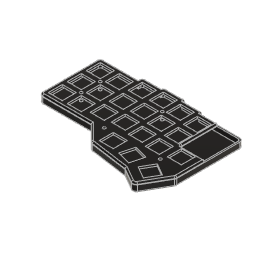
case-compact (Autodesk Fusion 360 design; units mm, degrees)
Autodesk Fusion 360 part; units mm, degrees
sketch "top_plate" plane through (0, 0, 0) normal (0, 0, 1) x (1, 0, 0)
  arc A0 (37, 57) -> (38, 58) centre (37, 58) ccw
  circle A1 centre (19, 38) radius 1.4
  circle A2 centre (76, 43) radius 1.4
  line L0 (117.5, 20.5) -> (131.5, 20.5)
  arc A3 (114, 24.5) -> (115.5, 23) centre (115.5, 24.5) ccw
  line L1 (95, 60) -> (95, 60)
  line L2 (95, 60) -> (95, 60)
  line L3 (96, 59) -> (112.5, 59)
  arc A4 (66.595, -15.7544) -> (67.4469, -16.1791) centre (67.6556, -14.6937) ccw
  line L4 (123.2697, -29.8066) -> (136.7998, -6.3468)
  arc A5 (106.318, -21.7524) -> (105.7767, -21.566) centre (105.568, -23.0514) ccw
  circle A6 centre (19, 19) radius 1.4
  line L5 (131.5, 20.5) -> (131.5, 6.5)
  line L6 (111.6878, -16.8122) -> (118.6878, -4.6878)
  line L7 (57, 62) -> (57, 62)
  arc A7 (0, 1.5) -> (1.5, 0) centre (1.5, 1.5) ccw
  line L8 (69.5, -13.5) -> (69.5, 0.5)
  line L9 (121.2203, -30.3563) -> (106.318, -21.7524)
  line L10 (118.6878, -4.6878) -> (130.8122, -11.6878)
  line L11 (58, 63) -> (75, 63)
  line L12 (38, 58) -> (38, 60)
  circle A8 centre (61, 0) radius 1.4
  line L13 (1.5, 57) -> (37, 57)
  line L14 (66.595, -15.7544) -> (51.2799, -0.4393)
  line L15 (93.5503, -0.9268) -> (107.0732, -4.5503)
  arc A9 (1.5, 57) -> (0, 55.5) centre (1.5, 55.5) ccw
  arc A10 (95, 60) -> (96, 59) centre (96, 60) ccw
  line L16 (117.5, 6.5) -> (117.5, 20.5)
  line L17 (135.5004, 23) -> (115.5, 23)
  line L18 (114, 24.5) -> (114, 57.5)
  arc A11 (121.2203, -30.3563) -> (123.2697, -29.8066) centre (121.9703, -29.0572) ccw
  arc A12 (136.7998, -6.3468) -> (137.0004, -5.5974) centre (135.5004, -5.5974) ccw
  arc A13 (76, 62) -> (75, 63) centre (75, 62) ccw
  line L19 (105.7767, -21.566) -> (67.4469, -16.1791)
  line L20 (123.8122, -23.8122) -> (111.6878, -16.8122)
  arc A14 (56, 61) -> (57, 62) centre (56, 62) ccw
  line L21 (0, 55.5) -> (0, 1.5)
  arc A15 (58, 63) -> (57, 62) centre (58, 62) ccw
  circle A16 centre (116, 1) radius 1.4
  arc A17 (39, 61) -> (38, 60) centre (39, 60) ccw
  line L22 (76, 62) -> (76, 62)
  line L23 (57, 62) -> (57, 62)
  line L24 (107.0732, -4.5503) -> (103.4497, -18.0732)
  line L25 (103.4497, -18.0732) -> (89.9268, -14.4497)
  line L26 (137.0004, 21.5) -> (137.0004, -5.5974)
  arc A18 (76, 62) -> (77, 61) centre (77, 62) ccw
  line L27 (89.9268, -14.4497) -> (93.5503, -0.9268)
  line L28 (76, 62) -> (76, 62)
  line L29 (1.5, 0) -> (50.2193, 0)
  line L30 (2.5, 40.5) -> (16.5, 40.5)
  line L31 (16.5, 40.5) -> (16.5, 54.5)
  line L32 (2.5, 54.5) -> (2.5, 40.5)
  line L33 (21.5, 2.5) -> (35.5, 2.5)
  line L34 (16.5, 35.5) -> (2.5, 35.5)
  line L35 (35.5, 2.5) -> (35.5, 16.5)
  line L36 (35.5, 21.5) -> (35.5, 35.5)
  line L37 (21.5, 16.5) -> (21.5, 2.5)
  line L38 (16.5, 54.5) -> (2.5, 54.5)
  line L39 (16.5, 21.5) -> (16.5, 35.5)
  line L40 (35.5, 16.5) -> (21.5, 16.5)
  line L41 (2.5, 35.5) -> (2.5, 21.5)
  line L42 (21.5, 21.5) -> (35.5, 21.5)
  line L43 (35.5, 35.5) -> (21.5, 35.5)
  line L44 (69.5, 0.5) -> (83.5, 0.5)
  line L45 (2.5, 21.5) -> (16.5, 21.5)
  line L46 (111.5, 42.5) -> (97.5, 42.5)
  line L47 (59.5, 8.5) -> (59.5, 22.5)
  line L48 (111.5, 37.5) -> (111.5, 23.5)
  line L49 (73.5, 46.5) -> (59.5, 46.5)
  line L50 (73.5, 41.5) -> (73.5, 27.5)
  line L51 (73.5, 22.5) -> (73.5, 8.5)
  line L52 (97.5, 18.5) -> (111.5, 18.5)
  line L53 (92.5, 39.5) -> (78.5, 39.5)
  line L54 (40.5, 20.5) -> (40.5, 6.5)
  line L55 (59.5, 27.5) -> (59.5, 41.5)
  line L56 (111.5, 4.5) -> (97.5, 4.5)
  line L57 (54.5, 44.5) -> (54.5, 58.5)
  line L58 (54.5, 20.5) -> (40.5, 20.5)
  line L59 (16.5, 2.5) -> (16.5, 16.5)
  line L60 (40.5, 39.5) -> (40.5, 25.5)
  line L61 (21.5, 40.5) -> (35.5, 40.5)
  line L62 (97.5, 56.5) -> (111.5, 56.5)
  line L63 (59.5, 60.5) -> (73.5, 60.5)
  line L64 (40.5, 44.5) -> (54.5, 44.5)
  line L65 (111.5, 56.5) -> (111.5, 42.5)
  line L66 (40.5, 25.5) -> (54.5, 25.5)
  line L67 (35.5, 40.5) -> (35.5, 54.5)
  arc A19 (95, 60) -> (94, 61) centre (94, 60) ccw
  line L68 (97.5, 23.5) -> (97.5, 37.5)
  line L69 (35.5, 54.5) -> (21.5, 54.5)
  line L70 (78.5, 39.5) -> (78.5, 25.5)
  line L71 (59.5, 22.5) -> (73.5, 22.5)
  line L72 (92.5, 44.5) -> (92.5, 58.5)
  line L73 (111.5, 23.5) -> (97.5, 23.5)
  line L74 (92.5, 25.5) -> (92.5, 39.5)
  line L75 (131.5, 6.5) -> (117.5, 6.5)
  line L76 (97.5, 4.5) -> (97.5, 18.5)
  line L77 (54.5, 58.5) -> (40.5, 58.5)
  line L78 (83.5, 0.5) -> (83.5, -13.5)
  line L79 (73.5, 8.5) -> (59.5, 8.5)
  line L80 (111.5, 18.5) -> (111.5, 4.5)
  line L81 (21.5, 35.5) -> (21.5, 21.5)
  line L82 (92.5, 6.5) -> (92.5, 20.5)
  line L83 (16.5, 16.5) -> (2.5, 16.5)
  line L84 (59.5, 41.5) -> (73.5, 41.5)
  line L85 (78.5, 6.5) -> (92.5, 6.5)
  line L86 (40.5, 58.5) -> (40.5, 44.5)
  line L87 (92.5, 20.5) -> (78.5, 20.5)
  line L88 (54.5, 25.5) -> (54.5, 39.5)
  line L89 (2.5, 16.5) -> (2.5, 2.5)
  line L90 (73.5, 27.5) -> (59.5, 27.5)
  line L91 (78.5, 25.5) -> (92.5, 25.5)
  line L92 (54.5, 6.5) -> (54.5, 20.5)
  line L93 (92.5, 58.5) -> (78.5, 58.5)
  arc A20 (137.0004, 21.5) -> (135.5004, 23) centre (135.5004, 21.5) ccw
  line L94 (130.8122, -11.6878) -> (123.8122, -23.8122)
  line L95 (39, 61) -> (56, 61)
  line L96 (77, 61) -> (94, 61)
  line L97 (40.5, 6.5) -> (54.5, 6.5)
  arc A21 (114, 57.5) -> (112.5, 59) centre (112.5, 57.5) ccw
  line L98 (97.5, 42.5) -> (97.5, 56.5)
  line L99 (78.5, 44.5) -> (92.5, 44.5)
  line L100 (21.5, 54.5) -> (21.5, 40.5)
  line L101 (73.5, 60.5) -> (73.5, 46.5)
  line L102 (59.5, 46.5) -> (59.5, 60.5)
  line L103 (54.5, 39.5) -> (40.5, 39.5)
  line L104 (78.5, 58.5) -> (78.5, 44.5)
  arc A22 (51.2799, -0.4393) -> (50.2193, 0) centre (50.2193, -1.5) ccw
  line L105 (97.5, 37.5) -> (111.5, 37.5)
  line L106 (83.5, -13.5) -> (69.5, -13.5)
  line L107 (2.5, 2.5) -> (16.5, 2.5)
  line L108 (78.5, 20.5) -> (78.5, 6.5)
  line L109 (77.8284, 63) -> (94, 63)
  arc A23 (96.8284, 61) -> (94, 63) centre (94, 60) ccw
  line L110 (96.8284, 61) -> (112.5, 61)
  line L111 (139.0004, 21.5) -> (139.0004, -5.5974)
  arc A24 (138.5323, -7.346) -> (139.0004, -5.5974) centre (135.5004, -5.5974) ccw
  line L112 (125.0022, -30.8058) -> (138.5323, -7.346)
  arc A25 (120.2203, -32.0883) -> (125.0022, -30.8058) centre (121.9703, -29.0572) ccw
  line L113 (120.2203, -32.0883) -> (105.4021, -23.5331)
  line L114 (105.4021, -23.5331) -> (67.1685, -18.1597)
  arc A26 (65.1808, -17.1686) -> (67.1685, -18.1597) centre (67.6556, -14.6937) ccw
  line L115 (65.1808, -17.1686) -> (50.0122, -2)
  line L116 (1.5, -2) -> (50.0122, -2)
  arc A27 (-2, 1.5) -> (1.5, -2) centre (1.5, 1.5) ccw
  line L117 (-2, 55.5) -> (-2, 1.5)
  arc A28 (1.5, 59) -> (-2, 55.5) centre (1.5, 55.5) ccw
  line L118 (1.5, 59) -> (36, 59)
  line L119 (36, 59) -> (36, 60)
  arc A29 (39, 63) -> (36, 60) centre (39, 60) ccw
  line L120 (39, 63) -> (55.1716, 63)
  arc A30 (58, 65) -> (55.1716, 63) centre (58, 62) ccw
  line L121 (58, 65) -> (75, 65)
  arc A31 (77.8284, 63) -> (75, 65) centre (75, 62) ccw
  line L122 (114, 57.5) -> (114, 59.5)
  line L123 (135.5004, 23) -> (137.5004, 23)
  arc A32 (114, 59.5) -> (112.5, 61) centre (112.5, 59.5) ccw
  arc A33 (139.0004, 21.5) -> (137.5004, 23) centre (137.5004, 21.5) ccw
  dimension "d10" = 1.5
  dimension "d11" = 1.5
  constraint tangent A21 L122
  constraint perpendicular L110 L122
  constraint parallel L96 L109
  constraint concentric A19 A23
  constraint parallel L3 L110
  constraint parallel L26 L111
  constraint concentric A12 A24
  constraint parallel L4 L112
  constraint concentric A11 A25
  constraint parallel L9 L113
  constraint parallel L19 L114
  constraint concentric A4 A26
  constraint parallel L14 L115
  constraint parallel L29 L116
  constraint concentric A7 A27
  constraint parallel L21 L117
  constraint concentric A9 A28
  constraint parallel L13 L118
  constraint parallel L12 L119
  constraint concentric A17 A29
  constraint parallel L95 L120
  constraint concentric A15 A30
  constraint parallel L11 L121
  constraint concentric A13 A31
  constraint tangent L109 A23
  constraint tangent A29 L120
  constraint tangent L111 A24
  constraint tangent A24 L112
  constraint tangent L112 A25
  constraint tangent A25 L113
  constraint tangent L114 A26
  constraint tangent A26 L115
  constraint tangent L116 A27
  constraint tangent A27 L117
  constraint tangent L117 A28
  constraint tangent A28 L118
  constraint tangent L119 A29
  constraint tangent A30 L121
  constraint tangent L121 A31
  constraint tangent A20 L123
  constraint perpendicular L111 L123
  constraint tangent L110 A32
  constraint tangent L122 A32
  constraint tangent L123 A33
  constraint tangent L111 A33
  measures "d10" radius of A32
  measures "d11" radius of A33
extrude "Extrude4" add sketch "top_plate" along normal blind 2 makes body 1
fillet "Fillet1" radius 1.5 27 edges at (18.75, 59, 2) (-0.9749, 57.9749, 2) (-2, 28.5, 2) (-0.9749, -0.9749, 2) (25.7561, -2, 2) (57.5965, -9.5843, 2) (66.0939, -17.826, 2) (86.2853, -20.8464, 2) (112.8112, -27.8107, 2) (122.8769, -32.4378, 2) (131.7673, -19.0759, 2) (138.8814, -6.5025, 2) (139.0004, 7.9513, 2) (138.5611, 22.5607, 2) (126.5002, 23, 2) (114.4393, 23.4393, 2) (114, 42, 2) (113.5607, 60.5607, 2) (104.6642, 61, 2) (95.7321, 62.4495, 2) (85.9142, 63, 2) (76.7321, 64.4495, 2) (66.5, 65, 2) (56.2679, 64.4495, 2) (47.0858, 63, 2) (36.8787, 62.1213, 2) (36, 59.5, 2) on bodies 1
sketch "bottom_plate" plane through (0, 0, 0) normal (0, 0, 1) x (1, 0, 0) in component "case-bottom"
  circle A0 centre (19, 38) radius 1.4
  circle A1 centre (61, 0) radius 1.4
  circle A2 centre (116, 1) radius 1.4
  arc A3 (56, 61) -> (57, 62) centre (56, 62) ccw
  circle A4 centre (76, 43) radius 1.4
  line L0 (121.2203, -30.3563) -> (106.318, -21.7524)
  line L1 (76, 62) -> (76, 62)
  line L2 (57, 62) -> (57, 62)
  line L3 (105.7767, -21.566) -> (67.4469, -16.1791)
  arc A5 (121.2203, -30.3563) -> (123.2697, -29.8066) centre (121.9703, -29.0572) ccw
  arc A6 (136.7994, -6.3479) -> (137, -5.5984) centre (135.5, -5.5984) ccw
  arc A7 (106.318, -21.7524) -> (105.7767, -21.566) centre (105.568, -23.0514) ccw
  arc A8 (76, 62) -> (75, 63) centre (75, 62) ccw
  line L4 (58, 63) -> (75, 63)
  arc A9 (95, 60) -> (96, 59) centre (96, 60) ccw
  arc A10 (0, 1.5) -> (1.5, 0) centre (1.5, 1.5) ccw
  arc A11 (51.2799, -0.4393) -> (50.2193, 0) centre (50.2193, -1.5) ccw
  line L5 (123.2697, -29.8066) -> (136.7994, -6.3479)
  arc A12 (37, 57) -> (38, 58) centre (37, 58) ccw
  arc A13 (66.595, -15.7544) -> (67.4469, -16.1791) centre (67.6556, -14.6937) ccw
  line L6 (1.5, 0) -> (50.2193, 0)
  line L7 (38, 58) -> (38, 60)
  line L8 (76, 62) -> (76, 62)
  line L9 (39, 61) -> (56, 61)
  arc A14 (39, 61) -> (38, 60) centre (39, 60) ccw
  line L10 (95, 60) -> (95, 60)
  line L11 (95, 60) -> (95, 60)
  line L12 (66.595, -15.7544) -> (51.2799, -0.4393)
  line L13 (0, 55.5) -> (0, 1.5)
  line L14 (1.5, 57) -> (37, 57)
  arc A15 (1.5, 57) -> (0, 55.5) centre (1.5, 55.5) ccw
  line L15 (77, 61) -> (94, 61)
  line L16 (57, 62) -> (57, 62)
  arc A16 (58, 63) -> (57, 62) centre (58, 62) ccw
  circle A17 centre (19, 19) radius 1.4
  line L17 (137, 57.5) -> (137, -5.5984)
  arc A18 (137, 57.5) -> (135.5, 59) centre (135.5, 57.5) ccw
  arc A19 (76, 62) -> (77, 61) centre (77, 62) ccw
  line L18 (95, 60) -> (95, 60)
  arc A20 (95, 60) -> (94, 61) centre (94, 60) ccw
  line L19 (96, 59) -> (135.5, 59)
  line L20 (96.8284, 61) -> (135.5, 61)
  arc A21 (139, 57.5) -> (135.5, 61) centre (135.5, 57.5) ccw
  line L21 (139, 57.5) -> (139, -5.5984)
  arc A22 (138.5319, -7.3471) -> (139, -5.5984) centre (135.5, -5.5984) ccw
  line L22 (125.0022, -30.8059) -> (138.5319, -7.3471)
  arc A23 (120.2203, -32.0883) -> (125.0022, -30.8059) centre (121.9703, -29.0572) ccw
  line L23 (120.2203, -32.0883) -> (105.4021, -23.5331)
  line L24 (105.4021, -23.5331) -> (67.1685, -18.1597)
  arc A24 (65.1808, -17.1686) -> (67.1685, -18.1597) centre (67.6556, -14.6937) ccw
  line L25 (65.1808, -17.1686) -> (50.0122, -2)
  line L26 (1.5, -2) -> (50.0122, -2)
  arc A25 (-2, 1.5) -> (1.5, -2) centre (1.5, 1.5) ccw
  line L27 (-2, 55.5) -> (-2, 1.5)
  arc A26 (1.5, 59) -> (-2, 55.5) centre (1.5, 55.5) ccw
  line L28 (1.5, 59) -> (36, 59)
  line L29 (36, 59) -> (36, 60)
  arc A27 (39, 63) -> (36, 60) centre (39, 60) ccw
  line L30 (39, 63) -> (55.1716, 63)
  arc A28 (58, 65) -> (55.1716, 63) centre (58, 62) ccw
  line L31 (58, 65) -> (75, 65)
  arc A29 (77.8284, 63) -> (75, 65) centre (75, 62) ccw
  line L32 (77.8284, 63) -> (94, 63)
  arc A30 (96.8284, 61) -> (94, 63) centre (94, 60) ccw
  arc A31 (95.5, 60) -> (96, 59.5) centre (96, 60) ccw
  line L33 (96, 59.5) -> (135.5, 59.5)
  arc A32 (137.5, 57.5) -> (135.5, 59.5) centre (135.5, 57.5) ccw
  line L34 (137.5, 57.5) -> (137.5, -5.5984)
  arc A33 (137.2325, -6.5977) -> (137.5, -5.5984) centre (135.5, -5.5984) ccw
  line L35 (123.7028, -30.0564) -> (137.2325, -6.5977)
  arc A34 (120.9703, -30.7893) -> (123.7028, -30.0564) centre (121.9703, -29.0572) ccw
  line L36 (120.9703, -30.7893) -> (106.068, -22.1854)
  arc A35 (106.068, -22.1854) -> (105.7071, -22.0612) centre (105.568, -23.0514) ccw
  line L37 (105.7071, -22.0612) -> (67.3773, -16.6743)
  arc A36 (66.2414, -16.1079) -> (67.3773, -16.6743) centre (67.6556, -14.6937) ccw
  line L38 (66.2414, -16.1079) -> (50.9264, -0.7929)
  arc A37 (50.9264, -0.7929) -> (50.2193, -0.5) centre (50.2193, -1.5) ccw
  line L39 (1.5, -0.5) -> (50.2193, -0.5)
  arc A38 (-0.5, 1.5) -> (1.5, -0.5) centre (1.5, 1.5) ccw
  line L40 (-0.5, 55.5) -> (-0.5, 1.5)
  arc A39 (1.5, 57.5) -> (-0.5, 55.5) centre (1.5, 55.5) ccw
  line L41 (1.5, 57.5) -> (37, 57.5)
  arc A40 (37, 57.5) -> (37.5, 58) centre (37, 58) ccw
  line L42 (37.5, 58) -> (37.5, 60)
  arc A41 (39, 61.5) -> (37.5, 60) centre (39, 60) ccw
  line L43 (39, 61.5) -> (56, 61.5)
  arc A42 (56, 61.5) -> (56.5, 62) centre (56, 62) ccw
  arc A43 (58, 63.5) -> (56.5, 62) centre (58, 62) ccw
  line L44 (58, 63.5) -> (75, 63.5)
  arc A44 (76.5, 62) -> (75, 63.5) centre (75, 62) ccw
  arc A45 (76.5, 62) -> (77, 61.5) centre (77, 62) ccw
  line L45 (77, 61.5) -> (94, 61.5)
  arc A46 (95.5, 60) -> (94, 61.5) centre (94, 60) ccw
  dimension "d14" = -2
  dimension "d24" = -0.5
extrude "Extrude4'" add sketch "bottom_plate" along normal blind 5 separate body contours L20 A21 L21 A22 L22 A23 L23 L24 A24 L25 L26 A25 L27 A26 L28 L29 A27 L30 A28 L31 A29 L32 A30 makes body 2 in component "case-bottom"
extrude "Extrude3" add sketch "bottom_plate" against normal blind 2 contours A3 L0 L3 A5 A6 A7 A8 L4 A9 A10 A11 L5 A12 A13 L6 L7 L9 A14 L12 L13 L14 A15 L15 A16 L17 A18 A19 A20 L19 | L20 A21 L21 A22 L22 A23 L23 L24 A24 L25 L26 A25 L27 A26 L28 L29 A27 L30 A28 L31 A29 L32 A30 | A31 L33 A32 L34 A33 L35 A34 L36 A35 L37 A36 L38 A37 L39 A38 L40 A39 L41 A40 L42 A41 L43 A42 A43 L44 A44 A45 L45 A46 bodies 2 in component "case-bottom"
move_body "Move1" bodies 1 to x (1, 0, 0) y (0, 1, 0) z (0, 0, 1) at (0, 0, 7)
move_body "Move2" bodies 1 to x (1, 0, 0) y (0, 1, 0) z (0, 0, 1) at (0, 0, -2)
fillet "Fillet2" radius 1.5 23 edges at (25.7561, -2, -2) (-0.9749, -0.9749, -2) (-2, 28.5, -2) (-0.9749, 57.9749, -2) (18.75, 59, -2) (86.2853, -20.8464, -2) (66.0939, -17.826, -2) (57.5965, -9.5843, -2) (116.1642, 61, -2) (137.9749, 59.9749, -2) (139, 25.9508, -2) (138.8809, -6.5035, -2) (131.767, -19.0765, -2) (122.8769, -32.4378, -2) (112.8112, -27.8107, -2) (85.9142, 63, -2) (95.7321, 62.4495, -2) (56.2679, 64.4495, -2) (66.5, 65, -2) (76.7321, 64.4495, -2) (36, 59.5, -2) (36.8787, 62.1213, -2) (47.0858, 63, -2) on bodies 2 in component "case-bottom"
sketch "Sketch5" plane through (0, 0, 5) normal (0, 0, 1) x (-1, 0, 0)
  arc A0 (-139, -57.5) -> (-135.5, -61) centre (-135.5, -57.5) ccw
  line L0 (-135.5, -61) -> (-96.8284, -61)
  arc A1 (-96.8284, -61) -> (-94, -63) centre (-94, -60) ccw
  line L1 (-94, -63) -> (-77.8284, -63)
  arc A2 (-77.8284, -63) -> (-75, -65) centre (-75, -62) ccw
  line L2 (-75, -65) -> (-58, -65)
  arc A3 (-58, -65) -> (-55.1716, -63) centre (-58, -62) ccw
  line L3 (-55.1716, -63) -> (-39, -63)
  arc A4 (-39, -63) -> (-36, -60) centre (-39, -60) ccw
  line L4 (-36, -60) -> (-36, -59)
  line L5 (-36, -59) -> (-1.5, -59)
  arc A5 (-1.5, -59) -> (2, -55.5) centre (-1.5, -55.5) ccw
  line L6 (2, -55.5) -> (2, -1.5)
  arc A6 (2, -1.5) -> (-1.5, 2) centre (-1.5, -1.5) ccw
  line L7 (-1.5, 2) -> (-50.0122, 2)
  line L8 (-50.0122, 2) -> (-65.1808, 17.1686)
  arc A7 (-65.1808, 17.1686) -> (-67.1685, 18.1597) centre (-67.6556, 14.6937) ccw
  line L9 (-67.1685, 18.1597) -> (-105.4021, 23.5331)
  line L10 (-105.4021, 23.5331) -> (-120.2203, 32.0883)
  arc A8 (-120.2203, 32.0883) -> (-125.0022, 30.8059) centre (-121.9703, 29.0572) ccw
  line L11 (-125.0022, 30.8059) -> (-138.5319, 7.3471)
  arc A9 (-138.5319, 7.3471) -> (-139, 5.5984) centre (-135.5, 5.5984) ccw
  line L12 (-139, 5.5984) -> (-139, -57.5)
  line L13 (-137, -57.5) -> (-137, -61)
  line L14 (-114, -59) -> (-135.5, -59)
  line L15 (-114, -59) -> (-114, -61)
  line L16 (-114, -61) -> (-137, -61)
  arc A10 (-95.5, -60) -> (-96, -59.5) centre (-96, -60) ccw
  line L17 (-96, -59.5) -> (-135.5, -59.5)
  arc A11 (-137.5, -57.5) -> (-135.5, -59.5) centre (-135.5, -57.5) ccw
  line L18 (-137.5, -57.5) -> (-137.5, 5.5984)
  arc A12 (-137.2325, 6.5977) -> (-137.5, 5.5984) centre (-135.5, 5.5984) ccw
  line L19 (-137.2325, 6.5977) -> (-123.7028, 30.0564)
  arc A13 (-120.9703, 30.7893) -> (-123.7028, 30.0564) centre (-121.9703, 29.0572) ccw
  line L20 (-120.9703, 30.7893) -> (-106.068, 22.1854)
  arc A14 (-106.068, 22.1854) -> (-105.7071, 22.0612) centre (-105.568, 23.0514) ccw
  line L21 (-105.7071, 22.0612) -> (-67.3773, 16.6743)
  arc A15 (-66.2414, 16.1079) -> (-67.3773, 16.6743) centre (-67.6556, 14.6937) ccw
  line L22 (-66.2414, 16.1079) -> (-50.9264, 0.7929)
  arc A16 (-50.9264, 0.7929) -> (-50.2193, 0.5) centre (-50.2193, 1.5) ccw
  line L23 (-50.2193, 0.5) -> (-1.5, 0.5)
  arc A17 (0.5, -1.5) -> (-1.5, 0.5) centre (-1.5, -1.5) ccw
  line L24 (0.5, -1.5) -> (0.5, -55.5)
  arc A18 (-1.5, -57.5) -> (0.5, -55.5) centre (-1.5, -55.5) ccw
  line L25 (-1.5, -57.5) -> (-37, -57.5)
  arc A19 (-37, -57.5) -> (-37.5, -58) centre (-37, -58) ccw
  line L26 (-37.5, -58) -> (-37.5, -60)
  arc A20 (-39, -61.5) -> (-37.5, -60) centre (-39, -60) ccw
  line L27 (-39, -61.5) -> (-56, -61.5)
  arc A21 (-56, -61.5) -> (-56.5, -62) centre (-56, -62) ccw
  arc A22 (-58, -63.5) -> (-56.5, -62) centre (-58, -62) ccw
  line L28 (-58, -63.5) -> (-75, -63.5)
  arc A23 (-76.5, -62) -> (-75, -63.5) centre (-75, -62) ccw
  arc A24 (-76.5, -62) -> (-77, -61.5) centre (-77, -62) ccw
  line L29 (-77, -61.5) -> (-94, -61.5)
  arc A25 (-95.5, -60) -> (-94, -61.5) centre (-94, -60) ccw
  constraint coincident L0 L15.end
  constraint perpendicular L0 L15
  constraint perpendicular L13 L16
extrude "Extrude5" cut sketch "Sketch5" against normal blind 2 contours A0 L13 L16 bodies 2 in component "case-bottom"
copy_body "Body->Comp1" bodies 1 removing the originals makes body 3 in component "case-top"
component "case-bottom" placed x (1, 0, 0) y (0, 1, 0) z (0, 0, 1) at (0, 0, 0)
component "case-top" placed x (1, 0, 0) y (0, 1, 0) z (0, 0, 1) at (0, 0, 0)
named bodies: "case-top", "case-bottom"
